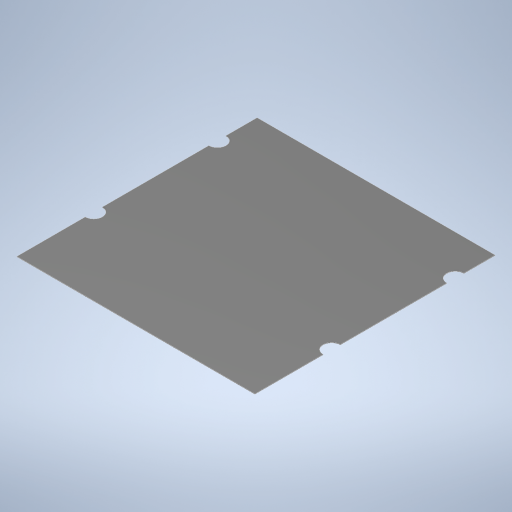
# Autodesk Inventor part: Coverplate Film
Saved by Autodesk Inventor 2023 (Build 270158000, 158)
## iProperties
Created: 2022-02-23
Part Number: Coverplate Film
Material: Thermoplastic Resin
Document SubType Name: Modeling
Designer: Caleb
Density: 1.28 g/cm^3
Appearance: Smooth - Black
Author: Caleb
Autodesk Inventor part; units mm, degrees
ref_plane "YZ Plane" through (0, 0, 0) normal (1, 0, 0) x (0, 1, 0)
ref_plane "XZ Plane" through (0, 0, 0) normal (0, 1, 0) x (-1, 0, 0)
ref_plane "XY Plane" through (0, 0, 0) normal (0, 0, 1) x (1, 0, 0)
sketch "Sketch1" plane through (0, 0, 0) normal (0, 1, 0) x (-1, 0, 0)
  line L0 (-20.8, -21) -> (20.8, -21)
  line L1 (20.8, -21) -> (20.8, 21)
  line L2 (20.8, 21) -> (-20.8, 21)
  line L3 (-20.8, 21) -> (-20.8, -21)
  line L4 (-20.8, -21) -> (20.8, 21) construction
  line L5 (20.8, -21) -> (-20.8, 21) construction
  point P0 (0, 0)
  dimension "d0" = 42
  dimension "d1" = 41.6
  constraints: 12 end point, 2 midpoint, 2 parallel, 1 horizontal, 1 perpendicular
  measures "d0" distance of L0.end L1.end
  measures "d1" distance of L1.end L2.end
extrude "Extrusion1" add sketch "Sketch1" along normal blind 0.08
sketch "Sketch2" plane through (0, 0.08, 0) normal (0, 1, 0) x (1, 0, 0)
  arc A0 (-20.8, 12.55) -> (-20.8, 15.55) centre (-20.8, 14.05) ccw
  line L0 (-20.8, 21) -> (-20.8, -21) projected
  line L1 (20.8, 21) -> (-20.8, 21) projected
  arc A1 (-20.8, -9.06) -> (-20.8, -6.06) centre (-20.8, -7.56) ccw
  line L2 (20.8, -21) -> (20.8, 21) projected
  arc A2 (20.8, 15.55) -> (20.8, 12.55) centre (20.8, 14.05) ccw
  arc A3 (20.8, -6.06) -> (20.8, -9.06) centre (20.8, -7.56) ccw
  point P0 (-20.8, 12.55)
  point P1 (20.8, -6.06)
  point P2 (20.8, -9.06)
  dimension "d5" = 1.5
  dimension "d8" = 3
  dimension "d9" = 6.95
  dimension "d10" = 1.5
  dimension "d11" = 1.5
  dimension "d12" = 1.5
  dimension "d13" = 28.56
  constraints: 8 point on circle, 8 point on line, 4 centre point, 2 horizontal alignment
  measures "d5" radius of A0
  measures "d8" distance of A0.start A0.end
  measures "d9" distance from line of L1 A0.centre
  measures "d10" radius of A1
  measures "d11" radius of A3
  measures "d12" radius of A2
  measures "d13" distance from line of L1 A1.centre
extrude "Extrusion2" cut sketch "Sketch2" against normal through all
equation "\"d10\" = d5"
equation "\"d11\" = d5"
equation "\"d12\" = d5"
body "Solid1"
